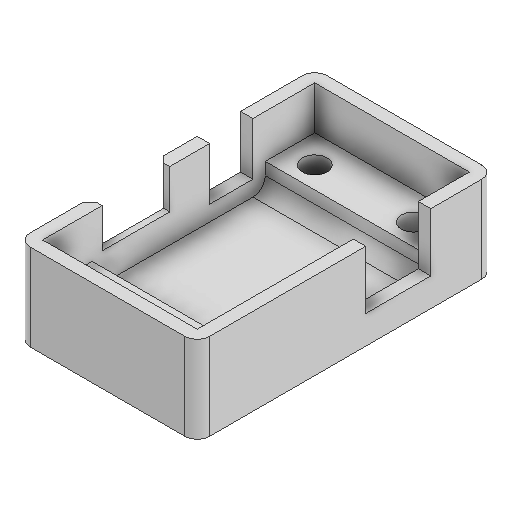
# Autodesk Inventor part: 3DP_ASA_Bias_Tee_Case_Bottom
Saved by Autodesk Inventor 2026.1 (Build 301233000, 233)
## iProperties
Created: 2025-06-27
Part Number: 3DP_ASA_Bias_Tee_Case_Bottom
Material: Generic
Document SubType Name: Modeling
Designer: User
Density: 1 g/cm^3
Appearance: Default
Author: User
Autodesk Inventor part; units mm, degrees
ref_plane "YZ Plane" through (0, 0, 0) normal (1, 0, 0) x (0, 1, 0)
ref_plane "XZ Plane" through (0, 0, 0) normal (0, 1, 0) x (-1, 0, 0)
ref_plane "XY Plane" through (0, 0, 0) normal (0, 0, 1) x (1, 0, 0)
sketch "Sketch1" plane through (0, 0, 0) normal (0, 1, 0) x (-1, 0, 0)
  line L0 (12, 21.5) -> (-12, 21.5)
  line L1 (-12, 21.5) -> (-12, -21.5)
  line L2 (-12, -21.5) -> (12, -21.5)
  line L3 (12, -21.5) -> (12, 21.5)
  line L4 (12.5, 22) -> (-12.5, 22)
  line L5 (-12.5, 22) -> (-12.5, -22)
  line L6 (-12.5, -22) -> (12.5, -22)
  line L7 (12.5, -22) -> (12.5, 22)
  line L8 (14.5, 24) -> (-14.5, 24)
  line L9 (-14.5, 24) -> (-14.5, -24)
  line L10 (-14.5, -24) -> (14.5, -24)
  line L11 (14.5, -24) -> (14.5, 24)
  circle A0 centre (8, 17.5) radius 2
  circle A1 centre (8, -17.5) radius 2
  circle A2 centre (-8, 17.5) radius 2
  circle A3 centre (-8, -17.5) radius 2
  point P0 (0, 0)
  dimension "d0" = 43
  dimension "d1" = 24
  dimension "d2" = 12
  dimension "d3" = 21.5
  dimension "d4" = 4
  dimension "d5" = 4
  dimension "d6" = 4
  dimension "d7" = 4
  dimension "d8" = 0.5
  dimension "d9" = 2
  dimension "d10" = 4
  dimension "d11" = 4
  dimension "d12" = 4
  dimension "d13" = 4
  constraints: 24 end point, 6 parallel, 4 centre point, 4 coincident, 3 perpendicular, 2 horizontal alignment, 2 vertical alignment, 1 horizontal, 6 other
  measures "d0" distance between parallel lines of L2 L0
  measures "d1" distance of L1.end L2.end
  measures "d2" distance from line of L3 point (0, 0)
  measures "d3" distance from line of L2 point (0, 0)
  measures "d4" distance from line of L0 point (8, 17.5)
  measures "d5" distance from line of L3 point (8, 17.5)
  measures "d6" distance from line of L1 point (-8, 17.5)
  measures "d7" distance from line of L2 point (8, -17.5)
  measures "d8" distance between parallel lines of L3 L7
  measures "d9" distance between parallel lines of L7 L11
  measures "d10" diameter of A0
  measures "d11" diameter of A1
  measures "d12" diameter of A2
  measures "d13" diameter of A3
extrude "Extrusion1" add sketch "Sketch1" against normal blind 7 contours L3 L2 L1 L0 | L7 L6 L5 L4 | L11 L10 L9 L8 | A0 | A1 | A2 | A3
extrude "Extrusion2" add sketch "Sketch1" along normal blind 7 contours L11 L10 L9 L8
extrude "Extrusion3" cut sketch "Sketch1" against normal blind 6 contours A0 | A1 | A2 | A3
sketch "Sketch2" plane through (0, 0, 0) normal (0, 1, 0) x (1, 0, 0)
  circle A0 centre (-8, -17.5) radius 2 projected
  circle A1 centre (8, 17.5) radius 2 projected
  circle A2 centre (8, -17.5) radius 2 projected
  circle A3 centre (-8, 17.5) radius 2 projected
  line L0 (-12.5, -22) -> (12.5, -22) projected
  line L1 (12.5, -22) -> (12.5, 22) projected
  line L2 (12.5, 22) -> (-12.5, 22) projected
  line L3 (-12.5, 22) -> (-12.5, -22) projected
  line L4 (-12.5, -14) -> (12.5, -14)
  line L5 (-12.5, 14) -> (12.5, 14)
  point P0 (0, 0)
  dimension "d20" = 8
  dimension "d21" = 8
  constraints: 4 end point, 4 point on line, 2 perpendicular
  measures "d20" distance between parallel lines of L2 L5
  measures "d21" distance between parallel lines of L0 L4
extrude "Extrusion4" cut sketch "Sketch2" against normal blind 4 contours L3 L5 L1 L4
sketch "Sketch3" plane through (14.5, -7, 24) normal (1, 0, 0) x (0, 0, -1)
  line L0 (0, 14) -> (0, 0) projected
  line L1 (48, 0) -> (0, 0) projected
  line L2 (48, 0) -> (48, 14) projected
  line L3 (0, 14) -> (48, 14) projected
  line L4 (27.74, 14) -> (27.74, 5.08)
  line L5 (27.74, 5.08) -> (37.26, 5.08)
  line L6 (37.26, 5.08) -> (37.26, 14)
  line L7 (37.76, 14) -> (37.76, 4.58)
  line L8 (37.76, 4.58) -> (27.24, 4.58)
  line L9 (27.24, 4.58) -> (27.24, 14)
  point P0 (24, 7)
  dimension "d24" = 9.52
  dimension "d25" = 27.74
  dimension "d26" = 8.92
  dimension "d27" = 0.5
  constraints: 12 end point, 3 perpendicular, 2 point on line, 1 vertical, 2 other
  measures "d24" distance between parallel lines of L6 L4
  measures "d25" distance between parallel lines of L0 L4
  measures "d26" distance between parallel lines of L3 L5
  measures "d27" distance between parallel lines of L5 L8
extrude "Extrusion5" cut sketch "Sketch3" against normal blind 7 contours L3 L4 L5 L6 L7 L8 L9 | L3 L6 L5 L4
sketch "Sketch4" plane through (-14.5, -7, -24) normal (-1, 0, 0) x (0, 0, 1)
  point P0 (24, 7)
sketch "Sketch5" plane through (-14.5, -7, -24) normal (-1, 0, 0) x (0, 0, 1)
  line L0 (0, 0) -> (0, 14) projected
  line L1 (48, 0) -> (0, 0) projected
  line L2 (48, 0) -> (48, 14) projected
  line L3 (0, 14) -> (48, 14) projected
  line L4 (35.38, 14) -> (35.38, 8.65)
  line L5 (35.38, 8.65) -> (26.44, 8.65)
  line L6 (26.44, 8.65) -> (26.44, 14)
  line L7 (25.44, 14) -> (25.44, 7.65)
  line L8 (25.44, 7.65) -> (36.38, 7.65)
  line L9 (36.38, 7.65) -> (36.38, 14)
  line L10 (12.5, 14) -> (12.5, 6)
  line L11 (12.5, 6) -> (18.5, 6)
  line L12 (18.5, 6) -> (18.5, 14)
  line L13 (12, 14) -> (12, 5.5)
  line L14 (12, 5.5) -> (19, 5.5)
  line L15 (19, 5.5) -> (19, 14)
  point P0 (24, 7)
  dimension "d30" = 8.94
  dimension "d31" = 12.62
  dimension "d32" = 5.35
  dimension "d33" = 1
  dimension "d34" = 6
  dimension "d35" = 12.5
  dimension "d36" = 8
  dimension "d37" = 0.5
  constraints: 24 end point, 6 perpendicular, 4 point on line, 2 vertical, 4 other
  measures "d30" distance between parallel lines of L6 L4
  measures "d31" distance between parallel lines of L2 L4
  measures "d32" distance between parallel lines of L3 L5
  measures "d33" distance between parallel lines of L5 L8
  measures "d34" distance between parallel lines of L12 L10
  measures "d35" distance between parallel lines of L0 L10
  measures "d36" distance between parallel lines of L11 L3
  measures "d37" distance between parallel lines of L10 L13
extrude "Extrusion6" cut sketch "Sketch5" against normal blind 7 contours L3 L10 L11 L12 L15 L14 L13 | L3 L12 L11 L10 | L9 L8 L7 L3 L6 L5 L4 | L4 L5 L6 L3
chamfer "Chamfer1" distance 1 angle 45 3 edges at (-14.5, 3.825, 12.38) (-14.5, 0.65, 6.91) (-14.5, 3.825, 1.44)
fillet "Fillet1" radius 2 4 edges at (-14.5, 0, -24) (14.5, 0, -24) (-14.5, 0, 24) (14.5, 0, 24)
fillet "Fillet2" radius 2 2 edges at (0, -4, 14) (0, -4, -14)
sketch "Sketch6" plane through (0, -7, 0) normal (0, -1, 0) x (1, 0, 0)
  line L0 (2.4904, 20.9325) -> (2.4904, -5.3505) construction
  line L1 (2.4904, -5.3505) -> (-0.6619, -5.3505) construction
  line L2 (-0.6619, -5.3505) -> (-0.6619, 20.9325) construction
  line L3 (-0.6619, 20.9325) -> (2.4904, 20.9325) construction
  line L4 (2.4065, 20.4218) -> (2.4065, 18.421)
  spline S0 degree 2 poles (2.4065, 18.421) (2.4065, 17.8265) (2.3075, 17.2435) (1.995, 16.7823) (1.4728, 16.4736) (1.1489, 16.4736) knots 0 0 0 1 2 3 4 4 4
  spline S1 degree 2 poles (1.1489, 16.4736) (0.7983, 16.4736) (0.2152, 16.8509) (0.0666, 17.1749) knots 0 0 0 1 2 2 2
  spline S2 degree 2 poles (0.0666, 17.1749) (-0.0668, 16.7175) (-0.707, 16.2297) (-1.1415, 16.2297) knots 0 0 0 1 2 2 2
  spline S3 degree 2 poles (-1.1415, 16.2297) (-1.4845, 16.2297) (-2.1285, 16.546) (-2.5134, 17.0986) (-2.5592, 17.4988) knots 0 0 0 1 2 3 3 3
  spline S4 degree 2 poles (-2.5592, 17.4988) (-2.5858, 17.7541) (-2.5935, 18.7183) knots 0 0 0 1 1 1
  line L5 (-2.5935, 18.7183) -> (-2.5935, 20.4218)
  line L6 (-2.5935, 20.4218) -> (2.4065, 20.4218)
  line L7 (-0.4098, 19.4119) -> (-1.7474, 19.4119)
  line L8 (-1.7474, 19.4119) -> (-1.7474, 18.4744)
  spline S5 degree 2 poles (-1.7474, 18.4744) (-1.7474, 17.9256) (-1.7169, 17.7808) knots 0 0 0 1 1 1
  spline S6 degree 2 poles (-1.7169, 17.7808) (-1.675, 17.556) (-1.3587, 17.2701) (-1.0919, 17.2701) knots 0 0 0 1 2 2 2
  spline S7 degree 2 poles (-1.0919, 17.2701) (-0.8671, 17.2701) (-0.5546, 17.4874) (-0.4098, 17.9028) (-0.4098, 18.5925) knots 0 0 0 1 2 3 3 3
  line L9 (-0.4098, 18.5925) -> (-0.4098, 19.4119)
  line L10 (1.5757, 19.4119) -> (0.421, 19.4119)
  line L11 (0.421, 19.4119) -> (0.421, 18.7488)
  spline S8 degree 2 poles (0.421, 18.7488) (0.421, 18.1581) (0.4363, 18.0133) knots 0 0 0 1 1 1
  spline S9 degree 2 poles (0.4363, 18.0133) (0.4706, 17.7541) (0.764, 17.4569) (1.0079, 17.4569) knots 0 0 0 1 2 2 2
  spline S10 degree 2 poles (1.0079, 17.4569) (1.2404, 17.4569) (1.5262, 17.7122) (1.5605, 17.9675) knots 0 0 0 1 2 2 2
  spline S11 degree 2 poles (1.5605, 17.9675) (1.5757, 18.1162) (1.5757, 18.8326) knots 0 0 0 1 1 1
  line L12 (1.5757, 18.8326) -> (1.5757, 19.4119)
  line L13 (-2.5935, 14.0651) -> (-0.4898, 14.0651)
  line L14 (-0.4898, 14.0651) -> (2.4065, 15.8944)
  line L15 (2.4065, 15.8944) -> (2.4065, 14.713)
  line L16 (2.4065, 14.713) -> (0.4248, 13.5316)
  line L17 (0.4248, 13.5316) -> (2.4065, 12.3807)
  line L18 (2.4065, 12.3807) -> (2.4065, 11.2145)
  line L19 (2.4065, 11.2145) -> (-0.4974, 13.0552)
  line L20 (-0.4974, 13.0552) -> (-2.5935, 13.0552)
  line L21 (-2.5935, 13.0552) -> (-2.5935, 14.0651)
  line L22 (-2.5935, 9.591) -> (1.5605, 9.591)
  line L23 (1.5605, 9.591) -> (1.5605, 11.0735)
  line L24 (1.5605, 11.0735) -> (2.4065, 11.0735)
  line L25 (2.4065, 11.0735) -> (2.4065, 7.1025)
  line L26 (2.4065, 7.1025) -> (1.5605, 7.1025)
  line L27 (1.5605, 7.1025) -> (1.5605, 8.5811)
  line L28 (1.5605, 8.5811) -> (-2.5935, 8.5811)
  line L29 (-2.5935, 8.5811) -> (-2.5935, 9.591)
  line L30 (-2.5935, 6.447) -> (2.4065, 6.447)
  line L31 (2.4065, 6.447) -> (2.4065, 2.7389)
  line L32 (2.4065, 2.7389) -> (1.5605, 2.7389)
  line L33 (1.5605, 2.7389) -> (1.5605, 5.4371)
  line L34 (1.5605, 5.4371) -> (0.4515, 5.4371)
  line L35 (0.4515, 5.4371) -> (0.4515, 2.9256)
  line L36 (0.4515, 2.9256) -> (-0.3945, 2.9256)
  line L37 (-0.3945, 2.9256) -> (-0.3945, 5.4371)
  line L38 (-0.3945, 5.4371) -> (-1.7474, 5.4371)
  line L39 (-1.7474, 5.4371) -> (-1.7474, 2.6436)
  line L40 (-1.7474, 2.6436) -> (-2.5935, 2.6436)
  line L41 (-2.5935, 2.6436) -> (-2.5935, 6.447)
  line L42 (-0.7528, -1.4113) -> (-1.0615, -2.3907)
  spline S12 degree 2 poles (-1.0615, -2.3907) (-1.8808, -2.1658) (-2.6773, -1.1178) (-2.6773, -0.3137) knots 0 0 0 1 2 2 2
  spline S13 degree 2 poles (-2.6773, -0.3137) (-2.6773, 0.681) (-1.3168, 1.9653) (-0.1392, 1.9653) knots 0 0 0 1 2 2 2
  spline S14 degree 2 poles (-0.1392, 1.9653) (1.1108, 1.9653) (2.4904, 0.6771) (2.4904, -0.3747) knots 0 0 0 1 2 2 2
  spline S15 degree 2 poles (2.4904, -0.3747) (2.4904, -1.2893) (1.9492, -1.8648) knots 0 0 0 1 1 1
  spline S16 degree 2 poles (1.9492, -1.8648) (1.6291, -2.204) (1.0308, -2.3754) knots 0 0 0 1 1 1
  line L43 (1.0308, -2.3754) -> (0.7907, -1.377)
  spline S17 degree 2 poles (0.7907, -1.377) (1.1794, -1.2893) (1.6291, -0.7253) (1.6291, -0.3251) knots 0 0 0 1 2 2 2
  spline S18 degree 2 poles (1.6291, -0.3251) (1.6291, 0.2313) (0.8326, 0.9249) (-0.063, 0.9249) knots 0 0 0 1 2 2 2
  spline S19 degree 2 poles (-0.063, 0.9249) (-1.0119, 0.9249) (-1.816, 0.2427) (-1.816, -0.3023) knots 0 0 0 1 2 2 2
  spline S20 degree 2 poles (-1.816, -0.3023) (-1.816, -0.7062) (-1.3015, -1.2855) (-0.7528, -1.4113) knots 0 0 0 1 2 2 2
  line L44 (-2.5935, -3.2596) -> (2.4065, -3.2596)
  line L45 (2.4065, -3.2596) -> (2.4065, -4.2695)
  line L46 (2.4065, -4.2695) -> (0.4401, -4.2695)
  line L47 (0.4401, -4.2695) -> (0.4401, -6.2474)
  line L48 (0.4401, -6.2474) -> (2.4065, -6.2474)
  line L49 (2.4065, -6.2474) -> (2.4065, -7.2573)
  line L50 (2.4065, -7.2573) -> (-2.5935, -7.2573)
  line L51 (-2.5935, -7.2573) -> (-2.5935, -6.2474)
  line L52 (-2.5935, -6.2474) -> (-0.406, -6.2474)
  line L53 (-0.406, -6.2474) -> (-0.406, -4.2695)
  line L54 (-0.406, -4.2695) -> (-2.5935, -4.2695)
  line L55 (-2.5935, -4.2695) -> (-2.5935, -3.2596)
  line L56 (-2.5935, -8.332) -> (2.3646, -8.332)
  line L57 (2.3646, -8.332) -> (2.3646, -9.3419)
  line L58 (2.3646, -9.3419) -> (-1.7474, -9.3419)
  line L59 (-1.7474, -9.3419) -> (-1.7474, -11.8533)
  line L60 (-1.7474, -11.8533) -> (-2.5935, -11.8533)
  line L61 (-2.5935, -11.8533) -> (-2.5935, -8.332)
  line L62 (-2.5935, -17.0782) -> (-2.5935, -15.9806)
  line L63 (-2.5935, -15.9806) -> (-1.4578, -15.5462)
  line L64 (-1.4578, -15.5462) -> (-1.4578, -13.5492)
  line L65 (-1.4578, -13.5492) -> (-2.5935, -13.1338)
  line L66 (-2.5935, -13.1338) -> (-2.5935, -12.0629)
  line L67 (-2.5935, -12.0629) -> (2.4065, -14.0065)
  line L68 (2.4065, -14.0065) -> (2.4065, -15.0812)
  line L69 (2.4065, -15.0812) -> (-2.5935, -17.0782)
  line L70 (-0.6118, -15.2222) -> (1.2404, -14.5325)
  line L71 (1.2404, -14.5325) -> (-0.6118, -13.8541)
  line L72 (-0.6118, -13.8541) -> (-0.6118, -15.2222)
  line L73 (2.4065, -17.6193) -> (2.4065, -19.6201)
  spline S21 degree 2 poles (2.4065, -19.6201) (2.4065, -20.2146) (2.3075, -20.7977) (1.995, -21.2588) (1.4728, -21.5675) (1.1489, -21.5675) knots 0 0 0 1 2 3 4 4 4
  spline S22 degree 2 poles (1.1489, -21.5675) (0.7983, -21.5675) (0.2152, -21.1902) (0.0666, -20.8663) knots 0 0 0 1 2 2 2
  spline S23 degree 2 poles (0.0666, -20.8663) (-0.0668, -21.3236) (-0.707, -21.8114) (-1.1415, -21.8114) knots 0 0 0 1 2 2 2
  spline S24 degree 2 poles (-1.1415, -21.8114) (-1.4845, -21.8114) (-2.1285, -21.4951) (-2.5134, -20.9425) (-2.5592, -20.5424) knots 0 0 0 1 2 3 3 3
  spline S25 degree 2 poles (-2.5592, -20.5424) (-2.5858, -20.287) (-2.5935, -19.3229) knots 0 0 0 1 1 1
  line L74 (-2.5935, -19.3229) -> (-2.5935, -17.6193)
  line L75 (-2.5935, -17.6193) -> (2.4065, -17.6193)
  line L76 (-0.4098, -18.6293) -> (-1.7474, -18.6293)
  line L77 (-1.7474, -18.6293) -> (-1.7474, -19.5668)
  spline S26 degree 2 poles (-1.7474, -19.5668) (-1.7474, -20.1155) (-1.7169, -20.2604) knots 0 0 0 1 1 1
  spline S27 degree 2 poles (-1.7169, -20.2604) (-1.675, -20.4852) (-1.3587, -20.771) (-1.0919, -20.771) knots 0 0 0 1 2 2 2
  spline S28 degree 2 poles (-1.0919, -20.771) (-0.8671, -20.771) (-0.5546, -20.5538) (-0.4098, -20.1384) (-0.4098, -19.4486) knots 0 0 0 1 2 3 3 3
  line L78 (-0.4098, -19.4486) -> (-0.4098, -18.6293)
  line L79 (1.5757, -18.6293) -> (0.421, -18.6293)
  line L80 (0.421, -18.6293) -> (0.421, -19.2924)
  spline S29 degree 2 poles (0.421, -19.2924) (0.421, -19.8831) (0.4363, -20.0279) knots 0 0 0 1 1 1
  spline S30 degree 2 poles (0.4363, -20.0279) (0.4706, -20.287) (0.764, -20.5843) (1.0079, -20.5843) knots 0 0 0 1 2 2 2
  spline S31 degree 2 poles (1.0079, -20.5843) (1.2404, -20.5843) (1.5262, -20.329) (1.5605, -20.0736) knots 0 0 0 1 2 2 2
  spline S32 degree 2 poles (1.5605, -20.0736) (1.5757, -19.925) (1.5757, -19.2085) knots 0 0 0 1 1 1
  line L81 (1.5757, -19.2085) -> (1.5757, -18.6293)
  point P0 (0, 0)
  constraints: 2 other
extrude "Extrusion7" cut sketch "Sketch6" against normal blind 0.2
equation "\"d2\" = 0.5 * d1"
equation "\"d3\" = 0.5 * d0"
equation "\"d5\" = d4"
equation "\"d6\" = d5"
equation "\"d7\" = d4"
body "Solid1"
